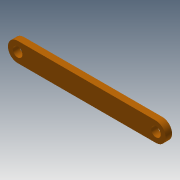
# Autodesk Inventor part: tahlo7
Saved by Autodesk Inventor 2015 (Build 190159000, 159)
## iProperties
Created: 2013-03-29
Part Number: tahlo7
Material: Generic
Document SubType Name: Modeling
Designer: idle-rug
Density: 1 g/cm^3
Appearance: Default
Author: idle-rug
Autodesk Inventor part; units mm, degrees
ref_plane "YZ Plane" through (0, 0, 0) normal (1, 0, 0) x (0, 1, 0)
ref_plane "XZ Plane" through (0, 0, 0) normal (0, 1, 0) x (-1, 0, 0)
ref_plane "XY Plane" through (0, 0, 0) normal (0, 0, 1) x (1, 0, 0)
sketch "Sketch1" plane through (0, 0, 0) normal (0, 1, 0) x (-1, 0, 0)
  line L0 (-21.5, -3) -> (21.5, -3)
  line L1 (21.5, -3) -> (21.5, 3)
  line L2 (21.5, 3) -> (-21.5, 3)
  line L3 (-21.5, 3) -> (-21.5, -3)
  line L4 (-21.5, -3) -> (21.5, 3) construction
  line L5 (21.5, -3) -> (-21.5, 3) construction
  circle A0 centre (21.5, 0) radius 3
  circle A1 centre (-21.5, 0) radius 3
  point P0 (0, 0)
  dimension "d0" = 43
  dimension "d1" = 6
  constraints: 12 end point, 4 midpoint, 2 parallel, 2 vertical alignment, 1 horizontal, 1 perpendicular, 4 other
  measures "d0" distance of L2.end L1.end
  measures "d1" distance of L1.end L0.end
extrude "Extrusion1" add sketch "Sketch1" along normal blind 2
sketch "Sketch2" plane through (0, 2, 0) normal (0, 1, 0) x (1, 0, 0)
  arc A0 (21.5, -3) -> (21.5, 3) centre (21.5, 0) ccw projected
  arc A1 (-21.5, 3) -> (-21.5, -3) centre (-21.5, 0) ccw projected
  circle A2 centre (-21.5, 0) radius 1.5
  circle A3 centre (21.5, 0) radius 1.5
  point P0 (0, 0)
  dimension "d5" = 3
  dimension "d6" = 3
  constraints: 2 centre point, 2 coincident
  measures "d5" diameter of A2
  measures "d6" diameter of A3
extrude "Extrusion2" cut sketch "Sketch2" against normal blind 2
sketch "Sketch3" plane through (0, 0, 0) normal (0, -1, 0) x (1, 0, 0)
  circle A0 centre (-21.5, 0) radius 1.5 projected
  circle A1 centre (21.5, 0) radius 1.5 projected
  arc A2 (21.5, -3) -> (21.5, 3) centre (21.5, 0) ccw projected
  arc A3 (-21.5, 3) -> (-21.5, -3) centre (-21.5, 0) ccw projected
  circle A4 centre (-21.5, 0) radius 0.05
  circle A5 centre (21.5, 0) radius 0.05
  point P0 (0, 0)
  dimension "d9" = 0.1
  dimension "d10" = 0.1
  constraints: 2 centre point, 2 coincident
  measures "d9" diameter of A4
  measures "d10" diameter of A5
extrude "Extrusion3" add sketch "Sketch3" against normal blind 2
sketch "Sketch4" plane through (0, 0, 0) normal (0, -1, 0) x (1, 0, 0)
  circle A0 centre (-21.5, 0) radius 0.05 projected
  circle A1 centre (21.5, 0) radius 0.05 projected
  arc A2 (21.5, -3) -> (21.5, 3) centre (21.5, 0) ccw projected
  arc A3 (-21.5, 3) -> (-21.5, -3) centre (-21.5, 0) ccw projected
  circle A4 centre (-21.5, 0) radius 1.5
  circle A5 centre (21.5, 0) radius 1.5
  point P0 (0, 0)
  dimension "d13" = 3
  dimension "d14" = 3
  constraints: 2 centre point, 2 coincident
  measures "d13" diameter of A4
  measures "d14" diameter of A5
extrude "Extrusion4" cut sketch "Sketch4" against normal blind 2
body "Solid1"
